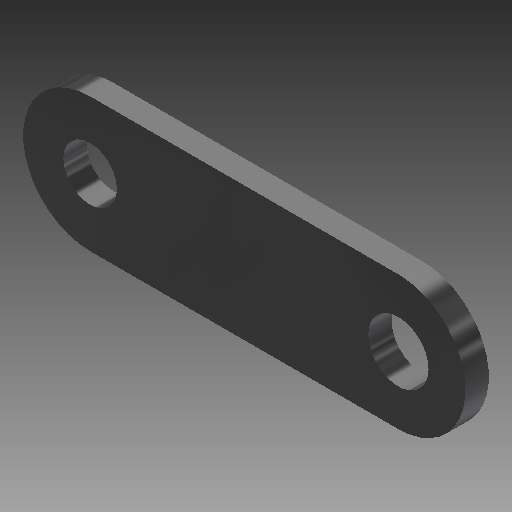
# Autodesk Inventor part: 201-12
Saved by Autodesk Inventor 2019 (Build 230136000, 136)
## iProperties
Company: Autodesk Inc.
Created: 2007-10-25
Part Number: 201-12
Document SubType Name: Modeling
Designer: Autodesk Inc.
Density: 7.85 g/cm^3
Mass: 30.7796 g
Surface Area: 29.6939 cm^2
Volume: 3.92097 cm^3
Material: Steel
Description: LINK PLATE
Appearance: Rubber - Black - Version 1.1
Component Category: Lower Component
Author: Inventor
Autodesk Inventor part; units mm, degrees
ref_plane "YZ Plane" through (0, 0, 0) normal (1, 0, 0) x (0, 1, 0)
ref_plane "XZ Plane" through (0, 0, 0) normal (0, 1, 0) x (-1, 0, 0)
ref_plane "XY Plane" through (0, 0, 0) normal (0, 0, 1) x (1, 0, 0)
sketch "Sketch1" plane through (0, 0, 0) normal (0, 0, 1) x (1, 0, 0)
  circle A0 centre (0, 0) radius 10
  line L0 (0, 0) -> (-46, 0) construction
  circle A1 centre (-46, 0) radius 10
  line L1 (-46, 10) -> (0, 10)
  line L2 (-46, -10) -> (0, -10)
  dimension "d0" = 20
  dimension "d1" = 20
  dimension "d2" = 46
  constraints: 6 end point, 4 point on circle, 4 tangent, 2 centre point, 2 coincident, 1 horizontal
  measures "d0" diameter of A1
  measures "d1" diameter of A0
  measures "d2" distance of point (0, 0) L0.end
extrude "Extrusion1" add sketch "Sketch1" along normal mid plane 3.5
hole "Hole3" at (-46, 0, 1.75) direction (0, 0, -1) diameter 8 end through all
hole "Hole4" at (0, 0, 1.75) direction (0, 0, -1) diameter 9 end through all
body "Solid1"
